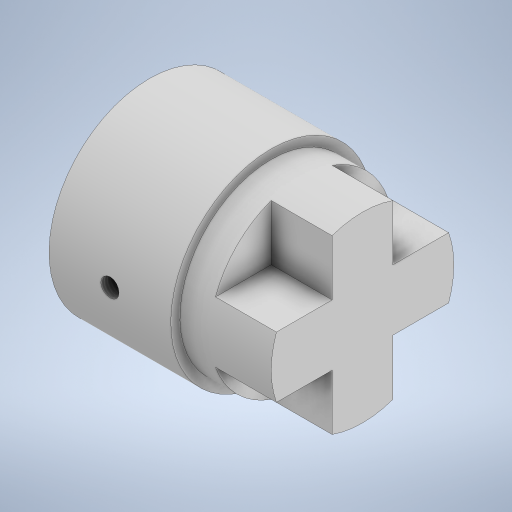
# Autodesk Inventor part: Втулка двигатель, вал
Saved by Autodesk Inventor 2023 (Build 270158000, 158)
## iProperties
Created: 2022-05-27
Part Number: Втулка двигатель, вал
Material: Типовые
Document SubType Name: Modeling
Designer: avkap
Density: 1 g/cm^3
Appearance: По умолчанию
Author: avkap
Autodesk Inventor part; units mm, degrees
ref_plane "YZ Plane" through (0, 0, 0) normal (1, 0, 0) x (0, 1, 0)
ref_plane "XZ Plane" through (0, 0, 0) normal (0, 1, 0) x (-1, 0, 0)
ref_plane "XY Plane" through (0, 0, 0) normal (0, 0, 1) x (1, 0, 0)
sketch "Эскиз1" plane through (0, 0, 0) normal (0, 0, 1) x (1, 0, 0)
  line L0 (0, 0) -> (20, 0)
  line L1 (0, 0) -> (0, 12.5)
  line L2 (0, 12.5) -> (0, 16.5)
  line L3 (0, 12.5) -> (20, 12.5)
  line L4 (20, 0) -> (20, 15)
  line L5 (20, 15) -> (35, 15)
  line L6 (35, 15) -> (35, 0)
  line L7 (35, 0) -> (20, 0)
  line L8 (0, 16.5) -> (20, 16.5)
  line L9 (20, 15) -> (20, 16.5)
  dimension "d0" = 20
  dimension "d1" = 12.5
  dimension "d2" = 4
  dimension "d5" = 15
  dimension "d6" = 15
  constraints: 20 end point, 5 perpendicular, 2 horizontal, 2 point on line, 1 collinear
  measures "d0" distance of L0.start L0.end
  measures "d1" distance of L0.start L1.end
  measures "d2" distance of L1.end L2.end
  measures "d5" distance of L4.end L5.end
  measures "d6" distance of L5.end L6.end
revolve "Вращение1" add sketch "Эскиз1" angle 360 about axis through (0, 0, 0) along (1, 0, 0) contours L4 L5 L6 L7 | L2 L8 L9 L4 L3
sketch "Эскиз2" plane through (0, 0, 0) normal (0, 0, 1) x (1, 0, 0)
  line L0 (0, 0) -> (10, 0)
  circle A0 centre (10, 0) radius 1.5
  dimension "d8" = 10
  dimension "d9" = 3
  constraints: 2 end point, 1 centre point, 1 coincident, 1 horizontal
  measures "d8" distance of L0.start L0.end
  measures "d9" diameter of A0
extrude "Выдавливание1" cut sketch "Эскиз2" along normal mid plane 40
thread "Резьба1" size "M3x0.5" class "6H" standard "ANSI Metric M Profile" full length
sketch "Эскиз3" plane through (35, 0, 0) normal (1, 0, 0) x (0, 0, -1)
  line L0 (0, 0) -> (-5, 0)
  line L1 (-5, 0) -> (-5, 20)
  line L2 (-5, 20) -> (5, 20)
  line L3 (5, 20) -> (5, -20)
  line L4 (5, -20) -> (-5, -20)
  line L5 (-5, -20) -> (-5, 0)
  circle A0 centre (0, 0) radius 15 projected
  line L6 (0, 0) -> (0, 5)
  line L7 (0, 5) -> (-20, 5)
  line L8 (-20, 5) -> (-20, -5)
  line L9 (-20, -5) -> (20, -5)
  line L10 (20, -5) -> (20, 5)
  line L11 (20, 5) -> (0, 5)
  point P0 (-5, -5)
  point P1 (-14.1421, -5)
  point P2 (-5, -14.1421)
  point P3 (14.1421, -5)
  point P4 (5, -5)
  point P5 (5, -14.1421)
  point P6 (5, 5)
  point P7 (14.1421, 5)
  point P8 (5, 14.1421)
  point P9 (-14.1421, 5)
  point P10 (-5, 5)
  point P11 (-5, 14.1421)
  dimension "d14" = 5
  dimension "d15" = 10
  dimension "d16" = 5
  dimension "d17" = 10
  constraints: 24 end point, 8 perpendicular, 2 collinear, 2 point on line, 1 horizontal, 1 vertical
  measures "d14" distance of L0.start L0.end
  measures "d15" distance of L1.end L2.end
  measures "d16" distance of L6.start L6.end
  measures "d17" distance of L7.end L8.end
extrude "Выдавливание2" cut sketch "Эскиз3" against normal blind 10 contours L7 A0 L1 | L5 A0 L9 | L3 A0 L11 | L9 A0 L3
